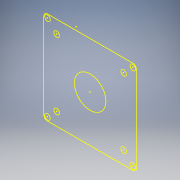
# Autodesk Inventor part: base_1
Saved by Autodesk Inventor 2019 (Build 230136000, 136)
## iProperties
Created: 2020-03-13
Part Number: base_1
Material: Generic
Document SubType Name: Modeling
Designer: Pulag
Density: 1 g/cm^3
Appearance: Default
Author: Pulag
Autodesk Inventor part; units mm, degrees
ref_plane "YZ Plane" through (0, 0, 0) normal (1, 0, 0) x (0, 1, 0)
ref_plane "XZ Plane" through (0, 0, 0) normal (0, 1, 0) x (-1, 0, 0)
ref_plane "XY Plane" through (0, 0, 0) normal (0, 0, 1) x (1, 0, 0)
sketch "Sketch1" plane through (0, 0, 0) normal (0, 0, 1) x (1, 0, 0)
  arc A0 (-17.7023, -49.8275) -> (-15.7023, -51.8275) centre (-15.7023, -49.8275) ccw projected
  line L0 (-15.7023, -51.8275) -> (30.2977, -51.8275) projected
  arc A1 (30.2977, -51.8275) -> (32.2977, -49.8275) centre (30.2977, -49.8275) ccw projected
  line L1 (32.2977, -49.8275) -> (32.2977, -3.8275) projected
  arc A2 (32.2977, -3.8275) -> (30.2977, -1.8275) centre (30.2977, -3.8275) ccw projected
  line L2 (30.2977, -1.8275) -> (-15.7023, -1.8275) projected
  arc A3 (-15.7023, -1.8275) -> (-17.7023, -3.8275) centre (-15.7023, -3.8275) ccw projected
  line L3 (-17.7023, -3.8275) -> (-17.7023, -49.8275) projected
  circle A4 centre (-15.7023, -3.8275) radius 1.5 projected
  circle A5 centre (-10.7525, -8.7773) radius 1.5 projected
  circle A6 centre (-10.7525, -44.8778) radius 1.5 projected
  circle A7 centre (-15.7023, -49.8275) radius 1.5 projected
  circle A8 centre (25.348, -44.8778) radius 1.5 projected
  circle A9 centre (30.2977, -49.8275) radius 1.5 projected
  circle A10 centre (25.348, -8.7773) radius 1.5 projected
  circle A11 centre (30.2977, -3.8275) radius 1.5 projected
  circle A12 centre (7.2977, -26.8275) radius 8.5 projected
  line L4 (-27.7023, 8.1725) -> (42.2977, 8.1725)
  line L5 (42.2977, 8.1725) -> (42.2977, -61.8275)
  line L6 (42.2977, -61.8275) -> (-27.7023, -61.8275)
  line L7 (-27.7023, -61.8275) -> (-27.7023, 8.1725)
  line L8 (-27.7023, 8.1725) -> (42.2977, -61.8275) construction
  line L9 (42.2977, 8.1725) -> (-27.7023, -61.8275) construction
  line L10 (42.2977, 8.1725) -> (-27.7023, 8.1725)
  line L11 (-27.7023, 8.1725) -> (-27.7023, 78.1725)
  line L12 (-27.7023, 78.1725) -> (42.2977, 78.1725)
  line L13 (42.2977, 78.1725) -> (42.2977, 8.1725)
  line L14 (11.2977, 68.1725) -> (38.2977, 68.1725)
  line L15 (38.2977, 68.1725) -> (38.2977, 18.1725)
  line L16 (38.2977, 18.1725) -> (11.2977, 18.1725)
  line L17 (11.2977, 18.1725) -> (11.2977, 68.1725)
  line L18 (11.2977, 68.1725) -> (38.2977, 18.1725) construction
  line L19 (38.2977, 68.1725) -> (11.2977, 18.1725) construction
  line L20 (-23.7023, 18.1725) -> (3.2977, 18.1725)
  line L21 (3.2977, 18.1725) -> (3.2977, 68.1725)
  line L22 (3.2977, 68.1725) -> (-23.7023, 68.1725)
  line L23 (-23.7023, 68.1725) -> (-23.7023, 18.1725)
  line L24 (-23.7023, 18.1725) -> (3.2977, 68.1725) construction
  line L25 (3.2977, 18.1725) -> (-23.7023, 68.1725) construction
  line L26 (4.7977, 69.6725) -> (4.7977, 16.6725)
  line L27 (-25.2023, 16.6725) -> (-25.2023, 69.6725)
  line L28 (-25.2023, 69.6725) -> (4.7977, 16.6725) construction
  line L29 (4.7977, 69.6725) -> (-25.2023, 16.6725) construction
  line L30 (39.7977, 69.6725) -> (39.7977, 16.6725)
  line L31 (9.7977, 16.6725) -> (9.7977, 69.6725)
  line L32 (9.7977, 69.6725) -> (39.7977, 16.6725) construction
  line L33 (39.7977, 69.6725) -> (9.7977, 16.6725) construction
  line L34 (38.2977, 68.1725) -> (38.2977, 69.6725)
  line L35 (11.2977, 68.1725) -> (11.2977, 69.6725)
  line L36 (11.2977, 18.1725) -> (11.2977, 16.6725)
  line L37 (38.2977, 18.1725) -> (38.2977, 16.6725)
  line L38 (3.2977, 69.6725) -> (3.2977, 68.1725)
  line L39 (3.2977, 18.1725) -> (3.2977, 16.6725)
  line L40 (-23.7023, 68.1725) -> (-23.7023, 69.6725)
  line L41 (-23.7023, 18.1725) -> (-23.7023, 16.6725)
  line L42 (-25.2023, 69.6725) -> (-23.7023, 69.6725)
  line L43 (3.2977, 69.6725) -> (4.7977, 69.6725)
  line L44 (4.7977, 16.6725) -> (3.2977, 16.6725)
  line L45 (-23.7023, 16.6725) -> (-25.2023, 16.6725)
  line L46 (39.7977, 16.6725) -> (38.2977, 16.6725)
  line L47 (11.2977, 16.6725) -> (9.7977, 16.6725)
  line L48 (9.7977, 69.6725) -> (11.2977, 69.6725)
  line L49 (38.2977, 69.6725) -> (39.7977, 69.6725)
  point P0 (0, 0)
  point P1 (24.7977, 43.1725)
  point P2 (-10.2023, 43.1725)
  dimension "d0" = 70
  dimension "d1" = 70
  dimension "d2" = 70
  dimension "d3" = 27
  dimension "d4" = 50
  dimension "d5" = 27
  dimension "d6" = 30
  dimension "d7" = 53
  dimension "d8" = 30
  dimension "d9" = 53
  constraints: 92 end point, 18 parallel, 14 perpendicular, 10 midpoint, 8 horizontal, 4 point on line, 1 collinear
  measures "d0" distance of L5.end L6.end
  measures "d1" distance of L4.end L5.end
  measures "d2" distance of L10.end L11.end
  measures "d3" distance of L15.end L16.end
  measures "d4" distance of L14.end L15.end
  measures "d5" distance of L22.end L21.end
  measures "d6" distance of L26.end L27.start
  measures "d7" distance of L26.start L26.end
  measures "d8" distance of L30.end L31.start
  measures "d9" distance of L30.start L30.end
sketch "Sketch2" plane through (0, 0, 0) normal (0, 0, 1) x (1, 0, 0)
  arc A0 (-17.7023, -49.8275) -> (-15.7023, -51.8275) centre (-15.7023, -49.8275) ccw
  line L0 (-15.7023, -51.8275) -> (30.2977, -51.8275)
  arc A1 (30.2977, -51.8275) -> (32.2977, -49.8275) centre (30.2977, -49.8275) ccw
  line L1 (32.2977, -49.8275) -> (32.2977, -3.8275)
  arc A2 (32.2977, -3.8275) -> (30.2977, -1.8275) centre (30.2977, -3.8275) ccw
  line L2 (30.2977, -1.8275) -> (-15.7023, -1.8275)
  arc A3 (-15.7023, -1.8275) -> (-17.7023, -3.8275) centre (-15.7023, -3.8275) ccw
  line L3 (-17.7023, -3.8275) -> (-17.7023, -49.8275)
  circle A4 centre (-15.7023, -3.8275) radius 1.5
  circle A5 centre (-10.7525, -8.7773) radius 1.5
  circle A6 centre (-10.7525, -44.8778) radius 1.5
  circle A7 centre (-15.7023, -49.8275) radius 1.5
  circle A8 centre (25.348, -44.8778) radius 1.5
  circle A9 centre (30.2977, -49.8275) radius 1.5
  circle A10 centre (25.348, -8.7773) radius 1.5
  circle A11 centre (30.2977, -3.8275) radius 1.5
  circle A12 centre (7.2977, -26.8275) radius 8.5
  line L4 (-27.7023, 8.1725) -> (42.2977, 8.1725)
  line L5 (42.2977, 8.1725) -> (42.2977, -61.8275)
  line L6 (42.2977, -61.8275) -> (-27.7023, -61.8275)
  line L7 (-27.7023, -61.8275) -> (-27.7023, 8.1725)
  line L8 (-27.7023, 8.1725) -> (42.2977, -61.8275) construction
  line L9 (42.2977, 8.1725) -> (-27.7023, -61.8275) construction
  line L10 (42.2977, 8.1725) -> (-27.7023, 8.1725)
  line L11 (-27.7023, 8.1725) -> (-27.7023, 78.1725)
  line L12 (-27.7023, 78.1725) -> (42.2977, 78.1725)
  line L13 (42.2977, 78.1725) -> (42.2977, 8.1725)
  line L14 (11.2977, 68.1725) -> (38.2977, 68.1725)
  line L15 (38.2977, 68.1725) -> (38.2977, 18.1725)
  line L16 (38.2977, 18.1725) -> (11.2977, 18.1725)
  line L17 (11.2977, 18.1725) -> (11.2977, 68.1725)
  line L18 (11.2977, 68.1725) -> (38.2977, 18.1725) construction
  line L19 (38.2977, 68.1725) -> (11.2977, 18.1725) construction
  line L20 (-23.7023, 18.1725) -> (3.2977, 18.1725)
  line L21 (3.2977, 18.1725) -> (3.2977, 68.1725)
  line L22 (3.2977, 68.1725) -> (-23.7023, 68.1725)
  line L23 (-23.7023, 68.1725) -> (-23.7023, 18.1725)
  line L24 (-23.7023, 18.1725) -> (3.2977, 68.1725) construction
  line L25 (3.2977, 18.1725) -> (-23.7023, 68.1725) construction
  line L26 (4.7977, 69.6725) -> (4.7977, 16.6725)
  line L27 (-25.2023, 16.6725) -> (-25.2023, 69.6725)
  line L28 (-25.2023, 69.6725) -> (4.7977, 16.6725) construction
  line L29 (4.7977, 69.6725) -> (-25.2023, 16.6725) construction
  line L30 (39.7977, 69.6725) -> (39.7977, 16.6725)
  line L31 (9.7977, 16.6725) -> (9.7977, 69.6725)
  line L32 (9.7977, 69.6725) -> (39.7977, 16.6725) construction
  line L33 (39.7977, 69.6725) -> (9.7977, 16.6725) construction
  line L34 (38.2977, 68.1725) -> (38.2977, 69.6725)
  line L35 (11.2977, 68.1725) -> (11.2977, 69.6725)
  line L36 (11.2977, 18.1725) -> (11.2977, 16.6725)
  line L37 (38.2977, 18.1725) -> (38.2977, 16.6725)
  line L38 (3.2977, 69.6725) -> (3.2977, 68.1725)
  line L39 (3.2977, 18.1725) -> (3.2977, 16.6725)
  line L40 (-23.7023, 68.1725) -> (-23.7023, 69.6725)
  line L41 (-23.7023, 18.1725) -> (-23.7023, 16.6725)
  line L42 (-25.2023, 69.6725) -> (-23.7023, 69.6725)
  line L43 (3.2977, 69.6725) -> (4.7977, 69.6725)
  line L44 (4.7977, 16.6725) -> (3.2977, 16.6725)
  line L45 (-23.7023, 16.6725) -> (-25.2023, 16.6725)
  line L46 (39.7977, 16.6725) -> (38.2977, 16.6725)
  line L47 (11.2977, 16.6725) -> (9.7977, 16.6725)
  line L48 (9.7977, 69.6725) -> (11.2977, 69.6725)
  line L49 (38.2977, 69.6725) -> (39.7977, 69.6725)
  point P0 (0, 0)
  point P1 (0, 0)
  point P2 (24.7977, 43.1725)
  point P3 (-10.2023, 43.1725)
  dimension "d10" = 70
  dimension "d11" = 70
  dimension "d12" = 70
  dimension "d13" = 27
  dimension "d14" = 50
  dimension "d15" = 27
  dimension "d16" = 30
  dimension "d17" = 53
  dimension "d18" = 30
  dimension "d19" = 53
  constraints: 100 end point, 18 parallel, 14 perpendicular, 13 centre point, 10 midpoint, 8 horizontal, 8 point on circle, 4 point on line, 1 collinear
  measures "d10" distance of L5.end L6.end
  measures "d11" distance of L4.end L5.end
  measures "d12" distance of L10.end L11.end
  measures "d13" distance of L15.end L16.end
  measures "d14" distance of L14.end L15.end
  measures "d15" distance of L22.end L21.end
  measures "d16" distance of L26.end L27.start
  measures "d17" distance of L26.start L26.end
  measures "d18" distance of L30.end L31.start
  measures "d19" distance of L30.start L30.end
extrude "Extrusion1" add sketch "Sketch1" against normal blind 3 contours L3 A3 L2 A2 L1 A1 L0 A0 | A4 | A5 | A6 | A7 | A8 | A9 | A10 | A11 | A12 | L11 L12 L13 L4 | L4 L5 L6 L7 | L14 L15 L16 L17 | L17 L36 L47 L31 L48 L35 | L34 L49 L30 L46 L37 L15 | L23 L22 L21 L20 | L41 L45 L27 L42 L40 L23 | L21 L38 L43 L26 L44 L39
extrude "Extrusion2" add sketch "Sketch2" along normal blind 8 contours L17 L36 L47 L31 L48 L35 | L34 L49 L30 L46 L37 L15 | L41 L45 L27 L42 L40 L23 | L21 L38 L43 L26 L44 L39
sketch "Sketch3" plane through (0, 0, 0) normal (0, 0, 1) x (1, 0, 0)
  arc A0 (-17.7023, -49.8275) -> (-15.7023, -51.8275) centre (-15.7023, -49.8275) ccw
  line L0 (-15.7023, -51.8275) -> (30.2977, -51.8275)
  arc A1 (30.2977, -51.8275) -> (32.2977, -49.8275) centre (30.2977, -49.8275) ccw
  line L1 (32.2977, -49.8275) -> (32.2977, -3.8275)
  arc A2 (32.2977, -3.8275) -> (30.2977, -1.8275) centre (30.2977, -3.8275) ccw
  line L2 (30.2977, -1.8275) -> (-15.7023, -1.8275)
  arc A3 (-15.7023, -1.8275) -> (-17.7023, -3.8275) centre (-15.7023, -3.8275) ccw
  line L3 (-17.7023, -3.8275) -> (-17.7023, -49.8275)
  circle A4 centre (-15.7023, -3.8275) radius 1.5
  circle A5 centre (-10.7525, -8.7773) radius 1.5
  circle A6 centre (-10.7525, -44.8778) radius 1.5
  circle A7 centre (-15.7023, -49.8275) radius 1.5
  circle A8 centre (25.348, -44.8778) radius 1.5
  circle A9 centre (30.2977, -49.8275) radius 1.5
  circle A10 centre (25.348, -8.7773) radius 1.5
  circle A11 centre (30.2977, -3.8275) radius 1.5
  circle A12 centre (7.2977, -26.8275) radius 8.5
  line L4 (-27.7023, 8.1725) -> (42.2977, 8.1725)
  line L5 (42.2977, 8.1725) -> (42.2977, -61.8275)
  line L6 (42.2977, -61.8275) -> (-27.7023, -61.8275)
  line L7 (-27.7023, -61.8275) -> (-27.7023, 8.1725)
  line L8 (-27.7023, 8.1725) -> (42.2977, -61.8275) construction
  line L9 (42.2977, 8.1725) -> (-27.7023, -61.8275) construction
  line L10 (42.2977, 8.1725) -> (-27.7023, 8.1725)
  line L11 (-27.7023, 8.1725) -> (-27.7023, 78.1725)
  line L12 (-27.7023, 78.1725) -> (42.2977, 78.1725)
  line L13 (42.2977, 78.1725) -> (42.2977, 8.1725)
  line L14 (11.2977, 68.1725) -> (38.2977, 68.1725)
  line L15 (38.2977, 68.1725) -> (38.2977, 18.1725)
  line L16 (38.2977, 18.1725) -> (11.2977, 18.1725)
  line L17 (11.2977, 18.1725) -> (11.2977, 68.1725)
  line L18 (11.2977, 68.1725) -> (38.2977, 18.1725) construction
  line L19 (38.2977, 68.1725) -> (11.2977, 18.1725) construction
  line L20 (-23.7023, 18.1725) -> (3.2977, 18.1725)
  line L21 (3.2977, 18.1725) -> (3.2977, 68.1725)
  line L22 (3.2977, 68.1725) -> (-23.7023, 68.1725)
  line L23 (-23.7023, 68.1725) -> (-23.7023, 18.1725)
  line L24 (-23.7023, 18.1725) -> (3.2977, 68.1725) construction
  line L25 (3.2977, 18.1725) -> (-23.7023, 68.1725) construction
  line L26 (4.7977, 69.6725) -> (4.7977, 16.6725)
  line L27 (-25.2023, 16.6725) -> (-25.2023, 69.6725)
  line L28 (-25.2023, 69.6725) -> (4.7977, 16.6725) construction
  line L29 (4.7977, 69.6725) -> (-25.2023, 16.6725) construction
  line L30 (39.7977, 69.6725) -> (39.7977, 16.6725)
  line L31 (9.7977, 16.6725) -> (9.7977, 69.6725)
  line L32 (9.7977, 69.6725) -> (39.7977, 16.6725) construction
  line L33 (39.7977, 69.6725) -> (9.7977, 16.6725) construction
  line L34 (38.2977, 68.1725) -> (38.2977, 69.6725)
  line L35 (11.2977, 68.1725) -> (11.2977, 69.6725)
  line L36 (11.2977, 18.1725) -> (11.2977, 16.6725)
  line L37 (38.2977, 18.1725) -> (38.2977, 16.6725)
  line L38 (3.2977, 69.6725) -> (3.2977, 68.1725)
  line L39 (3.2977, 18.1725) -> (3.2977, 16.6725)
  line L40 (-23.7023, 68.1725) -> (-23.7023, 69.6725)
  line L41 (-23.7023, 18.1725) -> (-23.7023, 16.6725)
  line L42 (-25.2023, 69.6725) -> (-23.7023, 69.6725)
  line L43 (3.2977, 69.6725) -> (4.7977, 69.6725)
  line L44 (4.7977, 16.6725) -> (3.2977, 16.6725)
  line L45 (-23.7023, 16.6725) -> (-25.2023, 16.6725)
  line L46 (39.7977, 16.6725) -> (38.2977, 16.6725)
  line L47 (11.2977, 16.6725) -> (9.7977, 16.6725)
  line L48 (9.7977, 69.6725) -> (11.2977, 69.6725)
  line L49 (38.2977, 69.6725) -> (39.7977, 69.6725)
  point P0 (0, 0)
  point P1 (0, 0)
  point P2 (0, 0)
  point P3 (24.7977, 43.1725)
  point P4 (-10.2023, 43.1725)
  dimension "d24" = 70
  dimension "d25" = 70
  dimension "d26" = 70
  dimension "d27" = 27
  dimension "d28" = 50
  dimension "d29" = 27
  dimension "d30" = 30
  dimension "d31" = 53
  dimension "d32" = 30
  dimension "d33" = 53
  constraints: 100 end point, 18 parallel, 14 perpendicular, 13 centre point, 10 midpoint, 8 horizontal, 8 point on circle, 4 point on line, 1 collinear
  measures "d24" distance of L5.end L6.end
  measures "d25" distance of L4.end L5.end
  measures "d26" distance of L10.end L11.end
  measures "d27" distance of L15.end L16.end
  measures "d28" distance of L14.end L15.end
  measures "d29" distance of L22.end L21.end
  measures "d30" distance of L26.end L27.start
  measures "d31" distance of L26.start L26.end
  measures "d32" distance of L30.end L31.start
  measures "d33" distance of L30.start L30.end
extrude "Extrusion3" add sketch "Sketch3" along normal blind 5 contours A12
body "Solid1"
